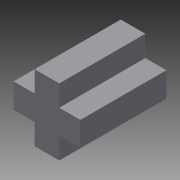
# Autodesk Inventor part: Croisillon
Saved by Autodesk Inventor 2015 (Build 190159000, 159)
## iProperties
Created: 2015-02-16
Part Number: Croisillon
Material: Générique
Document SubType Name: Modeling
Designer: informatique
Density: 1 g/cm^3
Appearance: Par défaut
Author: informatique
Autodesk Inventor part; units mm, degrees
ref_plane "YZ Plane" through (0, 0, 0) normal (1, 0, 0) x (0, 1, 0)
ref_plane "XZ Plane" through (0, 0, 0) normal (0, 1, 0) x (-1, 0, 0)
ref_plane "XY Plane" through (0, 0, 0) normal (0, 0, 1) x (1, 0, 0)
sketch "Esquisse1" plane through (0, 0, 0) normal (0, 1, 0) x (-1, 0, 0)
  line L0 (0.3187, 0.4542) -> (-0.3813, 0.4542)
  line L1 (-0.3813, 0.4542) -> (-0.3813, -1.4458)
  line L2 (-0.3813, -1.4458) -> (0.3187, -1.4458)
  line L3 (0.3187, -1.4458) -> (0.3187, 0.4542)
  line L4 (0.9187, -0.8458) -> (-0.9813, -0.8458)
  line L5 (-0.9813, -0.8458) -> (-0.9813, -0.1458)
  line L6 (-0.9813, -0.1458) -> (0.9187, -0.1458)
  line L7 (0.9187, -0.1458) -> (0.9187, -0.8458)
  point P0 (0, 0)
  dimension "d0" = 0.7
  dimension "d1" = 0.7
  dimension "d2" = 1.9
  dimension "d3" = 1.9
  dimension "d4" = 0.6
  dimension "d5" = 0.6
  constraints: 16 end point, 4 parallel, 2 horizontal, 2 perpendicular
  measures "d0" distance of L6.end L4.start
  measures "d1" distance of L1.end L2.end
  measures "d2" distance of L0.end L1.end
  measures "d3" distance of L4.start L4.end
  measures "d4" distance between parallel lines of L4 L2
  measures "d5" distance between parallel lines of L3 L7
extrude "Extrusion1" add sketch "Esquisse1" against normal blind 20.45
